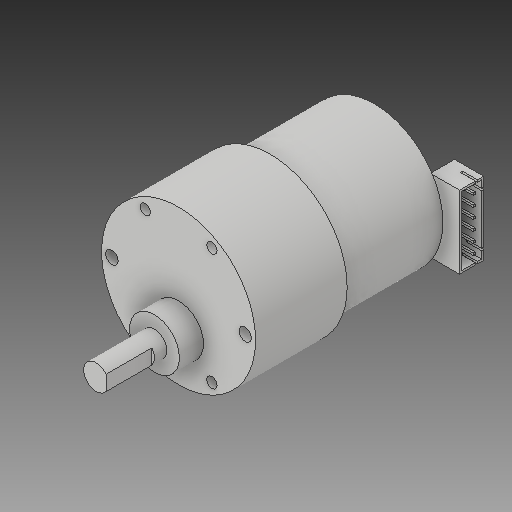
# Autodesk Inventor part: Motor
Saved by Autodesk Inventor 2018 (Build 220112000, 112)
## iProperties
Created: 2021-05-01
Part Number: Motor
Material: Generic
Document SubType Name: Modeling
Designer: dangl
Density: 1 g/cm^3
Appearance: Default
Author: dangl
Autodesk Inventor part; units mm, degrees
ref_plane "YZ Plane" through (0, 0, 0) normal (1, 0, 0) x (0, 1, 0)
ref_plane "XZ Plane" through (0, 0, 0) normal (0, 1, 0) x (-1, 0, 0)
ref_plane "XY Plane" through (0, 0, 0) normal (0, 0, 1) x (1, 0, 0)
sketch "Sketch1" plane through (0, 0, 0) normal (0, 0, 1) x (1, 0, 0)
  circle A0 centre (0, 0) radius 18.5
  dimension "d0" = 37
  constraints: 1 centre point, 1 coincident
  measures "d0" diameter of A0
extrude "Extrusion1" add sketch "Sketch1" against normal blind 22
sketch "Sketch2" plane through (0, 0, -22) normal (0, 0, -1) x (-1, 0, 0)
  circle A0 centre (0, 0) radius 18.5 projected
  circle A1 centre (0, 0) radius 16.5
  dimension "d3" = 33
  constraints: 1 centre point, 1 coincident
  measures "d3" diameter of A1
extrude "Extrusion2" add sketch "Sketch2" along normal blind 25 contours A1
sketch "Sketch3" plane through (0, 0, -47) normal (0, 0, -1) x (-1, 0, 0)
  circle A0 centre (0, 0) radius 18.5 projected
  circle A1 centre (0, 0) radius 7
  dimension "d6" = 14
  constraints: 1 centre point, 1 coincident
  measures "d6" diameter of A1
extrude "Extrusion3" add sketch "Sketch3" along normal blind 6.5 contours A1
sketch "Sketch4" plane through (0, 0, -53.5) normal (0, 0, -1) x (-1, 0, 0)
  circle A0 centre (0, 0) radius 1
  dimension "d9" = 2
  constraints: 1 centre point, 1 coincident
  measures "d9" diameter of A0
extrude "Extrusion4" add sketch "Sketch4" along normal blind 1.5
sketch "Sketch5" plane through (0, 0, -47) normal (0, 0, -1) x (-1, 0, 0)
  line L0 (-20.5, -8.75) -> (-13.5, -8.75)
  line L1 (-13.5, -8.75) -> (-13.5, 8.75)
  line L2 (-13.5, 8.75) -> (-20.5, 8.75)
  line L3 (-20.5, 8.75) -> (-20.5, -8.75)
  circle A0 centre (0, 0) radius 16.5 projected
  dimension "d12" = 17.5
  dimension "d13" = 7
  dimension "d14" = 8.75
  dimension "d15" = 37
  constraints: 8 end point, 2 parallel, 1 horizontal, 1 perpendicular
  measures "d12" distance of L2.end L0.start
  measures "d13" distance of L1.end L2.end
  measures "d14" distance from line of point (0, 0) L2
extrude "Extrusion5" add sketch "Sketch5" along normal blind 5.8 contours L3 L2 A0 L0 | A0 L2 L1 L0 picked at (-14.4657, -0.6136)
sketch "Sketch6" plane through (20.5, -8.75, -47) normal (1, 0, 0) x (0, 0, -1)
  line L0 (5.3, 17) -> (0.5, 17)
  line L1 (0.5, 17) -> (0.5, 0.5)
  line L2 (0.5, 0.5) -> (5.3, 0.5)
  line L3 (5.3, 0.5) -> (5.3, 17)
  line L4 (0, 17.5) -> (5.8, 17.5) projected
  line L5 (5.8, 17.5) -> (5.8, 0) projected
  line L6 (0, 0) -> (5.8, 0) projected
  line L7 (0, 17.5) -> (0, 0) projected
  line L8 (3.8, 15.25) -> (3.3, 15.25)
  line L9 (3.3, 15.25) -> (3.3, 14.75)
  line L10 (3.3, 14.75) -> (3.8, 14.75)
  line L11 (3.8, 14.75) -> (3.8, 15.25)
  line L12 (3.8, 12.75) -> (3.3, 12.75)
  line L13 (3.8, 12.25) -> (3.8, 12.75)
  line L14 (3.3, 12.25) -> (3.8, 12.25)
  line L15 (3.3, 12.75) -> (3.3, 12.25)
  line L16 (3.8, 10.25) -> (3.3, 10.25)
  line L17 (3.8, 9.75) -> (3.8, 10.25)
  line L18 (3.3, 9.75) -> (3.8, 9.75)
  line L19 (3.3, 10.25) -> (3.3, 9.75)
  line L20 (3.8, 7.75) -> (3.3, 7.75)
  line L21 (3.8, 7.25) -> (3.8, 7.75)
  line L22 (3.3, 7.25) -> (3.8, 7.25)
  line L23 (3.3, 7.75) -> (3.3, 7.25)
  line L24 (3.8, 5.25) -> (3.3, 5.25)
  line L25 (3.8, 4.75) -> (3.8, 5.25)
  line L26 (3.3, 4.75) -> (3.8, 4.75)
  line L27 (3.3, 5.25) -> (3.3, 4.75)
  line L28 (3.8, 2.75) -> (3.3, 2.75)
  line L29 (3.8, 2.25) -> (3.8, 2.75)
  line L30 (3.3, 2.25) -> (3.8, 2.25)
  line L31 (3.3, 2.75) -> (3.3, 2.25)
  line L32 (0, 17.5) -> (5.8, 17.5) projected
  line L33 (4.3185, 17) -> (3.8, 17)
  line L34 (3.8, 17) -> (3.8, 17.5)
  line L35 (3.8, 17.5) -> (4.3185, 17.5)
  line L36 (4.3185, 17.5) -> (4.3185, 17)
  line L37 (3.8, 0.5) -> (4.3185, 0.5)
  line L38 (4.3185, 0.5) -> (4.3185, 0)
  line L39 (4.3185, 0) -> (3.8, 0)
  line L40 (3.8, 0) -> (3.8, 0.5)
  line L41 (5.8, 15.25) -> (5.3, 15.25)
  line L42 (5.3, 15.25) -> (5.3, 14.75)
  line L43 (5.3, 14.75) -> (5.8, 14.75)
  line L44 (5.8, 14.75) -> (5.8, 15.25)
  line L45 (5.8, 2.75) -> (5.3, 2.75)
  line L46 (5.3, 2.75) -> (5.3, 2.25)
  line L47 (5.3, 2.25) -> (5.8, 2.25)
  line L48 (5.8, 2.25) -> (5.8, 2.75)
  point P0 (-47, 8.75)
  dimension "d18" = 0.5
  dimension "d19" = 0.5
  dimension "d20" = 0.5
  dimension "d21" = 0.5
  dimension "d22" = 0.5
  dimension "d23" = 0.5
  dimension "d26" = 2.5
  dimension "d31" = 1.5
  dimension "d32" = 1.75
  constraints: 88 end point, 12 parallel, 10 point on line, 6 horizontal, 6 perpendicular, 1 vertical, 40 other
  measures "d18" distance between parallel lines of L4 L0
  measures "d19" distance between parallel lines of L5 L3
  measures "d20" distance between parallel lines of L6 L2
  measures "d21" distance between parallel lines of L7 L1
  measures "d22" distance of L10.end L8.start
  measures "d23" distance of L9.end L10.end
  measures "d26" distance of L8.start L12.start
  measures "d31" distance between parallel lines of L3 L11
  measures "d32" distance between parallel lines of L0 L8
extrude "Extrusion6" cut sketch "Sketch6" against normal blind 5.5 contours L3 L2 L1 L0
extrude "Extrusion7" cut sketch "Sketch6" against normal blind 3.6 contours L0 L34 L4 L36 | L41 L5 L43 L3 | L45 L5 L47 L3 | L2 L38 L6 L40
sketch "Sketch7" plane through (0, 0, 0) normal (0, 0, 1) x (1, 0, 0)
  circle A0 centre (-8, 14) radius 1.25 projected
  circle A1 centre (-16, 0) radius 1.5 projected
  circle A2 centre (-8, -14) radius 1.25 projected
  circle A3 centre (8, -14) radius 1.25 projected
  circle A4 centre (16, 0) radius 1.5 projected
  circle A5 centre (8, 14) radius 1.25 projected
  circle A6 centre (0, -7) radius 6
  point P0 (0, 0)
  dimension "d37" = 12
  dimension "d38" = 7
  constraints: 1 centre point
  measures "d37" diameter of A6
  measures "d38" distance of A6.centre point (0, 0)
extrude "Extrusion8" add sketch "Sketch7" along normal blind 5.8 contours A6
sketch "Sketch8" plane through (0, -7, 5.8) normal (0, 0, 1) x (1, 0, 0)
  circle A0 centre (0, 7) radius 7 projected
  circle A1 centre (0, 0) radius 3
  dimension "d41" = 6
  constraints: 1 centre point, 1 vertical alignment, 1 other
  measures "d41" diameter of A1
extrude "Extrusion9" add sketch "Sketch8" along normal blind 14 contours A1 A0 | A0 A1 picked at (-0.8611, 0.9867) picked at (-1.0544, -0.7781)
sketch "Sketch9" plane through (0, -7, 19.8) normal (0, 0, 1) x (1, 0, 0)
  line L0 (2.4, 2.1786) -> (4.1019, 2.1786)
  line L1 (4.1019, 2.1786) -> (4.1019, -2.6301)
  line L2 (4.1019, -2.6301) -> (2.4, -2.6301)
  line L3 (2.4, -2.6301) -> (2.4, 2.1786)
  circle A0 centre (0, 0) radius 3 projected
  point P0 (0, 7)
  dimension "d44" = 5.4
  constraints: 8 end point, 2 parallel, 1 horizontal, 1 perpendicular
extrude "Extrusion10" cut sketch "Sketch9" against normal blind 11 contours L0 L1 L2 L3 A0 | A0 L3 picked at (2.5094, 0.416)
extrude "Extrusion11" cut sketch "Sketch7" against normal blind 10 contours A0 | A1 | A2 | A3 | A4 | A5
equation "\"d14\" = 0.5 * d12"
body "Solid1"
